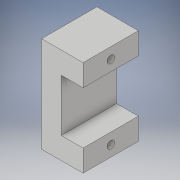
# Autodesk Inventor part: LidarV4MountBack
Saved by Autodesk Inventor 2019 (Build 230136000, 136)
## iProperties
Created: 2020-08-15
Part Number: LidarV4MountBack
Material: Generic
Document SubType Name: Modeling
Designer: james
Density: 1 g/cm^3
Appearance: Default
Author: james
Autodesk Inventor part; units mm, degrees
ref_plane "YZ Plane" through (0, 0, 0) normal (1, 0, 0) x (0, 1, 0)
ref_plane "XZ Plane" through (0, 0, 0) normal (0, 1, 0) x (-1, 0, 0)
ref_plane "XY Plane" through (0, 0, 0) normal (0, 0, 1) x (1, 0, 0)
sketch "Sketch1" plane through (0, 0, 0) normal (1, 0, 0) x (0, 1, 0)
  line L0 (22.6064, 29.4791) -> (-21.3864, 29.4791)
  line L1 (-21.3864, 29.4791) -> (-21.3864, 4.0791)
  line L2 (-21.3864, 4.0791) -> (22.6064, 4.0791)
  line L3 (22.6064, 4.0791) -> (22.6064, 29.4791)
  point P0 (0, 0)
  dimension "d0" = 43.9928
  dimension "d1" = 25.4
  constraints: 8 end point, 2 parallel, 1 horizontal, 1 perpendicular
  measures "d0" distance between parallel lines of L1 L3
  measures "d1" distance of L2.end L0.start
extrude "Extrusion1" add sketch "Sketch1" along normal blind 19.05
sketch "Sketch2" plane through (19.05, 0, 0) normal (1, 0, 0) x (0, 0, -1)
  line L0 (-29.4791, 22.6064) -> (-29.4791, -21.3864) projected
  line L1 (-29.4791, -21.3864) -> (-4.0791, -21.3864) projected
  line L2 (-4.0791, 22.6064) -> (-29.4791, 22.6064) projected
  point P0 (0, 0)
  point P1 (-16.7791, 17.6064)
  point P2 (-16.7791, -16.3864)
  dimension "d4" = 0
  dimension "d5" = 12.7
  dimension "d6" = 5
  dimension "d7" = 5
  measures "d4" horizontal distance of point (-16.779, -16.386) point (-16.779, 17.606)
  measures "d5" distance from line of L0 point (-16.779, -16.386)
  measures "d6" distance from line of L1 point (-16.779, -16.386)
  measures "d7" distance from line of L2 point (-16.779, 17.606)
hole "Hole1" at (19.05, 17.6064, 16.7791) at (19.05, -16.3864, 16.7791) direction (-1, 0, 0) diameter 3.4036 end through all clearance for "Flat Head Machine Screw" size "M3" standard "Ansi Metric M Profile"
sketch "Sketch3" plane through (0, -21.3864, 29.4791) normal (0, 0, 1) x (1, 0, 0)
  line L0 (19.05, 10) -> (9.05, 10)
  line L1 (9.05, 10) -> (9.05, 33.9928)
  line L2 (9.05, 33.9928) -> (19.05, 33.9928)
  line L3 (19.05, 33.9928) -> (19.05, 10)
  line L4 (19.05, 43.9928) -> (19.05, 0) projected
  line L5 (0, 43.9928) -> (19.05, 43.9928) projected
  line L6 (0, 0) -> (19.05, 0) projected
  point P0 (0, 21.3864)
  dimension "d15" = 0
  dimension "d16" = 10
  dimension "d17" = 10
  dimension "d18" = 10
  constraints: 8 end point, 2 parallel, 1 horizontal, 1 perpendicular
  measures "d15" distance between parallel lines of L4 L3
  measures "d16" distance between parallel lines of L5 L2
  measures "d17" distance between parallel lines of L6 L0
  measures "d18" distance between parallel lines of L3 L1
extrude "Extrusion2" cut sketch "Sketch3" against normal blind 60.325
body "Solid1"
